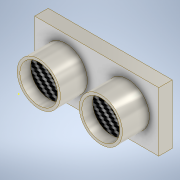
# Autodesk Inventor part: ir sensor
Saved by Autodesk Inventor 2021 (Build 250183000, 183)
## iProperties
Created: 2021-07-13
Part Number: ir sensor
Material: Titanium
Document SubType Name: Modeling
Designer: VK
Density: 4.51 g/cm^3
Appearance: Titanium
Author: VK
Autodesk Inventor part; units mm, degrees
ref_plane "YZ Plane" through (0, 0, 0) normal (1, 0, 0) x (0, 1, 0)
ref_plane "XZ Plane" through (0, 0, 0) normal (0, 1, 0) x (-1, 0, 0)
ref_plane "XY Plane" through (0, 0, 0) normal (0, 0, 1) x (1, 0, 0)
sketch "Sketch1" plane through (0, 0, 0) normal (0, 0, 1) x (1, 0, 0)
  line L0 (0, 0) -> (46, 0)
  line L1 (46, 0) -> (46, 22)
  line L2 (46, 22) -> (0, 22)
  line L3 (0, 22) -> (0, 0)
  dimension "d0" = 46
  dimension "d1" = 22
  constraints: 8 end point, 2 parallel, 1 horizontal, 1 perpendicular
  measures "d0" distance of L2.end L1.end
  measures "d1" distance of L1.end L0.end
extrude "Extrusion1" add sketch "Sketch1" along normal blind 5
sketch "Sketch2" plane through (0, 0, 5) normal (0, 0, 1) x (1, 0, 0)
  line L0 (0, 0) -> (46, 0) projected
  line L1 (46, 0) -> (46, 22) projected
  circle A0 centre (11.5, 11) radius 8
  circle A1 centre (34.5, 11) radius 8
  point P0 (23, 0)
  point P1 (23, 21.9141)
  point P2 (23, 11)
  point P3 (0, 11)
  point P4 (46, 11)
  dimension "d4" = 16
  dimension "d5" = 16
  constraints: 2 centre point, 2 coincident, 2 midpoint
  measures "d4" diameter of A0
  measures "d5" diameter of A1
extrude "Extrusion2" add sketch "Sketch2" along normal blind 10
sketch "Sketch3" plane through (11.5, 11, 15) normal (0, 0, 1) x (1, 0, 0)
  circle A0 centre (0, 0) radius 7
  point P0 (-11.5, -11)
  dimension "d8" = 14
  constraints: 1 centre point
  measures "d8" diameter of A0
sketch "Sketch4" plane through (34.5, 11, 15) normal (0, 0, 1) x (1, 0, 0)
  circle A0 centre (0, 0) radius 7
  point P0 (-34.5, -11)
  dimension "d9" = 14
  constraints: 1 centre point
  measures "d9" diameter of A0
extrude "Extrusion3" cut sketch "Sketch3" against normal blind 4
extrude "Extrusion4" cut sketch "Sketch4" against normal blind 4
sketch "Sketch5" plane through (11.5, 11, 11) normal (0, 0, 1) x (1, 0, 0)
  point P0 (-11.5, -11)
sketch "Sketch6" plane through (0, 0, 5) normal (0, 0, 1) x (1, 0, 0)
  point P0 (0, 0)
body "Solid1"
